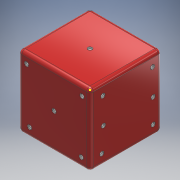
# Autodesk Inventor part: Part2
Saved by Autodesk Inventor 2018 (Build 220112000, 112)
## iProperties
Created: 2018-04-20
Part Number: Part2
Material: Generic
Document SubType Name: Modeling
Designer: dilan haddad
Density: 1 g/cm^3
Appearance: Default
Author: dilan haddad
Autodesk Inventor part; units mm, degrees
ref_plane "YZ Plane" through (0, 0, 0) normal (1, 0, 0) x (0, 1, 0)
ref_plane "XZ Plane" through (0, 0, 0) normal (0, 1, 0) x (-1, 0, 0)
ref_plane "XY Plane" through (0, 0, 0) normal (0, 0, 1) x (1, 0, 0)
sketch "Sketch1" plane through (0, 0, 0) normal (0, 1, 0) x (-1, 0, 0)
  line L0 (0, 0) -> (10, 0)
  line L1 (10, 0) -> (10, 10)
  line L2 (10, 10) -> (0, 10)
  line L3 (0, 10) -> (0, 0)
  dimension "d0" = 10
  dimension "d1" = 10
  constraints: 8 end point, 2 parallel, 1 horizontal, 1 perpendicular
  measures "d0" distance of L2.end L1.end
  measures "d1" distance of L1.end L0.end
extrude "Extrusion1" add sketch "Sketch1" along normal blind 10
fillet "Fillet1" radius 0.5 1 edges at (-5, 10, 10)
fillet "Fillet2" radius 0.5 3 edges at (0, 10, 4.75) (0, 9.8536, 9.8536) (0, 4.75, 10)
fillet "Fillet3" radius 0.5 3 edges at (-5.25, 0, 10) (-0.1464, 0, 9.8536) (0, 0, 4.75)
fillet "Fillet4" radius 0.5 5 edges at (-10, 10, 4.75) (-10, 9.8536, 9.8536) (-10, 5, 10) (-10, 0.1464, 9.8536) (-10, 0, 4.75)
fillet "Fillet5" radius 0.5 8 edges at (-5, 10, 0) (-9.8536, 9.8536, 0) (-10, 5, 0) (-9.8536, 0.1464, 0) (-5, 0, 0) (-0.1464, 0.1464, 0) (0, 5, 0) (-0.1464, 9.8536, 0)
sketch "Sketch2" plane through (-0.5, 0.5, 10) normal (0, 0, 1) x (1, 0, 0)
  line L0 (-9, 0) -> (0, 0) projected
  line L1 (0, 9) -> (-9, 9) projected
  circle A0 centre (-4.5, 4.5004) radius 0.3149
  point P0 (0.5, -0.5)
  constraints: 1 centre point
hole "Hole1" at (-5, 5.0004, 10) direction (0, 0, -1) diameter 0.5 depth 0.2 tip angle 118
sketch "Sketch3" plane through (-0.5, 0.5, 10) normal (0, 0, 1) x (1, 0, 0)
  point P0 (0.5, -0.5)
sketch "Sketch4" plane through (0, 10, 0) normal (0, 1, 0) x (1, 0, 0)
  circle A0 centre (-1.7172, -8.1418) radius 0.25
  circle A1 centre (-7.9617, -1.9694) radius 0.25
  point P0 (0, 0)
  dimension "d16" = 0.5
  dimension "d17" = 0.5
  constraints: 2 centre point
  measures "d16" diameter of A0
  measures "d17" diameter of A1
hole "Hole2" at (-1.7172, 10, 8.1418) direction (0, -1, 0) diameter 0.5 depth 0.2 tip angle 118
sketch "Sketch5" plane through (0, 10, 0) normal (0, 1, 0) x (1, 0, 0)
  circle A0 centre (-8.1941, -1.7607) radius 0.25
  point P0 (0, 0)
  dimension "d25" = 0.5
  constraints: 1 centre point
  measures "d25" diameter of A0
hole "Hole3" at (-8.1941, 10, 1.7607) direction (0, -1, 0) diameter 0.5 depth 0.2 tip angle 118
sketch "Sketch6" plane through (-10, 0.5, 9.5) normal (-1, 0, 0) x (0, 0, 1)
  circle A0 centre (-8.0109, 1.0971) radius 0.25
  circle A1 centre (-4.8407, 4.5) radius 0.25
  point P0 (-9.5, -0.5)
  dimension "d33" = 0.5
  dimension "d34" = 0.5
  constraints: 2 centre point
  measures "d33" diameter of A0
  measures "d34" diameter of A1
hole "Hole4" at (-10, 5, 4.6593) direction (1, 0, 0) diameter 0.5 depth 0.2 tip angle 118
sketch "Sketch7" plane through (-10, 0.5, 9.5) normal (-1, 0, 0) x (0, 0, 1)
  circle A0 centre (-8.0109, 1.1452) radius 0.25
  point P0 (-9.5, -0.5)
  dimension "d42" = 0.5
  constraints: 1 centre point
  measures "d42" diameter of A0
hole "Hole5" at (-10, 1.6452, 1.4891) direction (1, 0, 0) diameter 0.5 depth 0.2 tip angle 118
sketch "Sketch8" plane through (-10, 0.5, 9.5) normal (-1, 0, 0) x (0, 0, 1)
  circle A0 centre (-1.094, 8.2303) radius 0.25
  point P0 (-9.5, -0.5)
  dimension "d50" = 0.5
  constraints: 1 centre point
  measures "d50" diameter of A0
hole "Hole6" at (-10, 8.7303, 8.406) direction (1, 0, 0) diameter 0.5 depth 0.2 tip angle 118
sketch "Sketch9" plane through (-0.5, 9.5, 0) normal (0, 0, -1) x (-1, 0, 0)
  circle A0 centre (0.929, -8.107) radius 0.25
  point P0 (-0.5, -9.5)
  dimension "d58" = 0.5
  constraints: 1 centre point
  measures "d58" diameter of A0
hole "Hole7" at (-1.429, 1.393, 0) direction (0, 0, 1) diameter 0.5 depth 0.2 tip angle 118
sketch "Sketch10" plane through (-0.5, 9.5, 0) normal (0, 0, -1) x (-1, 0, 0)
  circle A0 centre (0.679, -0.9018) radius 0.25
  point P0 (-0.5, -9.5)
  dimension "d66" = 0.5
  constraints: 1 centre point
  measures "d66" diameter of A0
hole "Hole8" at (-1.179, 8.5982, 0) direction (0, 0, 1) diameter 0.5 depth 0.2 tip angle 118
sketch "Sketch11" plane through (-0.5, 9.5, 0) normal (0, 0, -1) x (-1, 0, 0)
  circle A0 centre (8.0381, -0.9018) radius 0.25
  point P0 (-0.5, -9.5)
  dimension "d74" = 0.5
  constraints: 1 centre point
  measures "d74" diameter of A0
hole "Hole9" at (-8.5381, 8.5982, 0) direction (0, 0, 1) diameter 0.5 depth 0.2 tip angle 118
sketch "Sketch12" plane through (-0.5, 9.5, 0) normal (0, 0, -1) x (-1, 0, 0)
  circle A0 centre (8.0381, -8.0109) radius 0.25
  point P0 (-0.5, -9.5)
  dimension "d28" = 3.023
  dimension "d82" = 0.5
  constraints: 1 centre point
  measures "d82" diameter of A0
hole "Hole10" at (-8.5381, 1.4891, 0) direction (0, 0, 1) diameter 0.5 depth 0.2 tip angle 118
sketch "Sketch13" plane through (0, 0.5, 9.5) normal (1, 0, 0) x (0, 0, -1)
  circle A0 centre (8.059, 8.3023) radius 0.25
  point P0 (9.5, -0.5)
  dimension "d90" = 0.5
  constraints: 1 centre point
  measures "d90" diameter of A0
hole "Hole11" at (0, 8.8023, 1.441) direction (-1, 0, 0) diameter 0.5 depth 0.2 tip angle 118
sketch "Sketch14" plane through (0, 0.5, 9.5) normal (1, 0, 0) x (0, 0, -1)
  circle A0 centre (8.0109, 1.1452) radius 0.25 projected
  circle A1 centre (8.0109, 1.1452) radius 0.25
  point P0 (9.5, -0.5)
  dimension "d98" = 0.5
  constraints: 1 centre point, 1 coincident
  measures "d98" diameter of A1
hole "Hole12" at (0, 1.6452, 1.4891) direction (-1, 0, 0) diameter 0.5 depth 0.2 tip angle 118
sketch "Sketch15" plane through (0, 0.5, 9.5) normal (1, 0, 0) x (0, 0, -1)
  circle A0 centre (4.7391, 8.3023) radius 0.25
  point P0 (9.5, -0.5)
  dimension "d106" = 0.5
  constraints: 1 centre point
  measures "d106" diameter of A0
hole "Hole13" at (0, 8.8023, 4.7609) direction (-1, 0, 0) diameter 0.5 depth 0.2 tip angle 118
sketch "Sketch16" plane through (0, 0.5, 9.5) normal (1, 0, 0) x (0, 0, -1)
  circle A0 centre (1.094, 8.2303) radius 0.25 projected
  circle A1 centre (1.094, 8.2303) radius 0.25
  point P0 (9.5, -0.5)
  dimension "d114" = 0.5
  constraints: 1 centre point, 1 coincident
  measures "d114" diameter of A1
hole "Hole14" at (0, 8.7303, 8.406) direction (-1, 0, 0) diameter 0.5 depth 0.2 tip angle 118
sketch "Sketch17" plane through (0, 0.5, 9.5) normal (1, 0, 0) x (0, 0, -1)
  circle A0 centre (4.7391, 1.3716) radius 0.25
  point P0 (9.5, -0.5)
  dimension "d122" = 0.5
  constraints: 1 centre point
  measures "d122" diameter of A0
hole "Hole15" at (0, 1.8716, 4.7609) direction (-1, 0, 0) diameter 0.5 depth 0.2 tip angle 118
sketch "Sketch18" plane through (0, 0.5, 9.5) normal (1, 0, 0) x (0, 0, -1)
  circle A0 centre (1.094, 1.299) radius 0.25
  point P0 (9.5, -0.5)
  dimension "d130" = 0.5
  constraints: 1 centre point
  measures "d130" diameter of A0
hole "Hole16" at (0, 1.799, 8.406) direction (-1, 0, 0) diameter 0.5 depth 0.2 tip angle 118
sketch "Sketch19" plane through (0, 0, 0) normal (0, -1, 0) x (1, 0, 0)
  circle A0 centre (-1.2129, 1.2969) radius 0.25
  point P0 (0, 0)
  dimension "d138" = 0.5
  constraints: 1 centre point
  measures "d138" diameter of A0
hole "Hole17" at (-1.2129, 0, 1.2969) direction (0, 1, 0) diameter 0.5 depth 0.2 tip angle 118
sketch "Sketch20" plane through (0, 0, 0) normal (0, -1, 0) x (1, 0, 0)
  circle A0 centre (-8.418, 1.2969) radius 0.25
  point P0 (0, 0)
  dimension "d146" = 0.5
  constraints: 1 centre point
  measures "d146" diameter of A0
hole "Hole18" at (-8.418, 0, 1.2969) direction (0, 1, 0) diameter 0.5 depth 0.2 tip angle 118
sketch "Sketch21" plane through (0, 0, 0) normal (0, -1, 0) x (1, 0, 0)
  circle A0 centre (-5.0076, 4.9716) radius 0.25
  point P0 (0, 0)
  dimension "d154" = 0.5
  constraints: 1 centre point
  measures "d154" diameter of A0
hole "Hole19" at (-5.0076, 0, 4.9716) direction (0, 1, 0) diameter 0.5 depth 0.2 tip angle 118
sketch "Sketch22" plane through (0, 0, 0) normal (0, -1, 0) x (1, 0, 0)
  circle A0 centre (-1.1168, 8.6942) radius 0.25
  point P0 (0, 0)
  dimension "d162" = 0.5
  constraints: 1 centre point
  measures "d162" diameter of A0
hole "Hole20" at (-1.1168, 0, 8.6942) direction (0, 1, 0) diameter 0.5 depth 0.2 tip angle 118
sketch "Sketch23" plane through (0, 0, 0) normal (0, -1, 0) x (1, 0, 0)
  circle A0 centre (-8.8503, 8.7183) radius 0.25
  point P0 (0, 0)
  dimension "d170" = 0.5
  constraints: 1 centre point
  measures "d170" diameter of A0
hole "Hole21" at (-8.8503, 0, 8.7183) direction (0, 1, 0) diameter 0.5 depth 0.2 tip angle 118
fillet "Fillet6" radius 0.05 1 edges at (0, 8.8023, 1.691)
fillet "Fillet7" radius 0.05 1 edges at (0, 8.8023, 5.0109)
fillet "Fillet8" radius 0.05 1 edges at (0, 1.6452, 1.7391)
fillet "Fillet9" radius 0.05 1 edges at (0, 1.8716, 5.0109)
fillet "Fillet10" radius 0.05 1 edges at (0, 1.799, 8.656)
fillet "Fillet11" radius 0.05 1 edges at (0, 8.7303, 8.656)
fillet "Fillet12" radius 0.05 1 edges at (-8.1941, 10, 1.5107)
fillet "Fillet13" radius 0.05 1 edges at (-1.7172, 10, 7.8918)
fillet "Fillet14" radius 0.05 1 edges at (-8.5381, 1.2391, 0)
fillet "Fillet15" radius 0.05 1 edges at (-8.5381, 8.3482, 0)
fillet "Fillet16" radius 0.05 1 edges at (-1.179, 8.3482, 0)
fillet "Fillet17" radius 0.05 1 edges at (-1.429, 1.143, 0)
fillet "Fillet18" radius 0.05 1 edges at (-1.2129, 0, 1.5469)
fillet "Fillet19" radius 0.05 1 edges at (-5.0076, 0, 5.2216)
fillet "Fillet20" radius 0.05 1 edges at (-1.1168, 0, 8.9442)
fillet "Fillet21" radius 0.05 1 edges at (-8.8503, 0, 8.9683)
fillet "Fillet22" radius 0.05 1 edges at (-8.418, 0, 1.5469)
fillet "Fillet23" radius 0.05 1 edges at (-10, 1.6452, 1.2391)
fillet "Fillet24" radius 0.05 1 edges at (-10, 5, 4.4093)
fillet "Fillet25" radius 0.05 1 edges at (-10, 8.7303, 8.156)
fillet "Fillet26" radius 0.05 1 edges at (-5, 5.2504, 10)
body "Solid1"
